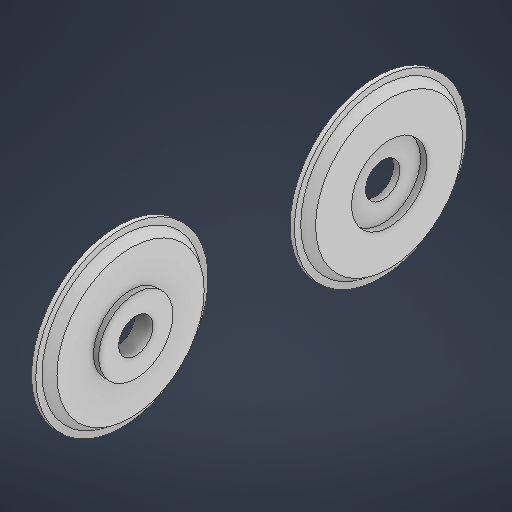
# Autodesk Inventor part: Polea_pulgar_falange1
Saved by Autodesk Inventor 2026.1 (Build 301233020, 233B)
## iProperties
Created: 2026-02-22
Part Number: Polea_pulgar_falange1
Material: Generic
Document SubType Name: Modeling
Designer: user
Density: 1 g/cm^3
Appearance: Default
Author: user
Autodesk Inventor part; units mm, degrees
ref_plane "XY Plane" through (0, 0, 0) normal (0, 0, 1) x (1, 0, 0)
sketch "Sketch1" plane through (0, 0, 0) normal (1, 0, 0) x (0, 1, 0)
  circle A0 centre (0, 0) radius 8.5399
  dimension "d0" = 17.0798
  constraints: 1 centre point, 1 coincident
  measures "d0" diameter of A0
extrude "Extrusion1" add sketch "Sketch1" along normal mid plane 2
sketch "Sketch2" plane through (-1, 0, 0) normal (-1, 0, 0) x (0, 0, 1)
  circle A0 centre (0, 0) radius 10
  dimension "d41" = 20
  constraints: 1 centre point, 1 coincident
  measures "d41" diameter of A0
extrude "Extrusion2" add sketch "Sketch2" along normal blind 0.5
sketch "Sketch3" plane through (-1.5, 0, 0) normal (-1, 0, 0) x (0, 0, 1)
  point P0 (0, 0)
sketch "Sketch5" plane through (0, 0, 0) normal (0, 1, 0) x (-1, 0, 0)
  circle A0 centre (0, -0.6447) radius 0.3263
  line L0 (-1.5, 0) -> (1.5, 0)
  circle A1 centre (0, 0.6447) radius 0.3263
  point P0 (0, 0)
  constraints: 2 centre point, 2 end point, 1 symmetric about line, 1 other
sketch "Sketch6" plane through (0, 0, 0) normal (0, 1, 0) x (-1, 0, 0)
  line L0 (1, -8.5399) -> (1, 8.5399) projected
  line L1 (1, -8.5399) -> (-1, -8.5399) projected
  line L2 (0, -8.5399) -> (1, -5.5929)
  line L3 (1, -10) -> (1, 10) projected
  line L4 (0, -8.5399) -> (-1, -9.2623)
  line L5 (-1, -9.2623) -> (-1, -8.5399)
  line L6 (1, -8.5399) -> (1, -9.2623)
  line L7 (-2.6263, 0) -> (3.0126, 0)
  line L8 (-1, -9.2623) -> (-1, -8.5399)
  line L9 (0, -8.5399) -> (1, -8.5399)
  point P0 (0, 0)
  constraints: 14 end point, 1 horizontal, 1 midpoint, 1 perpendicular, 1 point on line
revolve "Revolution1" add sketch "Sketch6" angle 360 about axis through (2.6263, 0, 0) along (-1, 0, 0) contours L4 L5 L1
mirror "Mirror3" about plane through (0, 0, 0) normal (1, 0, 0) of "Revolution1"
sketch "Sketch7" plane through (0, 0, 0) normal (0, 1, 0) x (-1, 0, 0)
  line L0 (-5.9098, -10.3165) -> (0, -10.3165)
  line L1 (0, -10.3165) -> (0, 11.166)
  line L2 (0, 11.166) -> (-5.9098, 11.166)
  line L3 (-5.9098, 11.166) -> (-5.9098, -10.3165)
  point P0 (0, 0)
  constraints: 8 end point, 2 parallel, 1 horizontal, 1 perpendicular
extrude "Extrusion6" cut sketch "Sketch7" along normal mid plane 24.5
sketch "Sketch8" plane through (0, 0, 0) normal (1, 0, 0) x (0, 1, 0)
  circle A0 centre (0, 0) radius 2
  dimension "d15" = 4
  constraints: 1 centre point, 1 coincident
  measures "d15" diameter of A0
extrude "Extrusion7" cut sketch "Sketch8" against normal through all
sketch "Sketch9" plane through (0, 0, 0) normal (1, 0, 0) x (0, 0, -1)
  circle A0 centre (0, 0) radius 4.374
  line L0 (1.4796, -4.1161) -> (1.4796, -1.3457)
  circle A1 centre (0, 0) radius 2 projected
  arc A2 (1.4796, -1.3457) -> (-1.4796, -1.3457) centre (0, 0) ccw
  line L1 (0.971, -8.4845) -> (0.971, 2) projected
  line L2 (-1.4796, -4.1161) -> (-1.4796, -1.3457)
  line L3 (-0.971, 2) -> (-0.971, -8.4845) projected
  point P0 (0.971, -4.7727)
  point P1 (0, 2)
  point P2 (0, 2)
  point P3 (-0.971, -4.7727)
  point P4 (-1.4796, -1.3457)
  point P5 (0.971, -7.875)
  point P6 (-0.971, -7.875)
  dimension "d22" = 0.5086
  dimension "d23" = 0.5086
  dimension "d36" = 8.7479
  constraints: 5 point on circle, 4 end point, 2 centre point, 2 coincident, 1 parallel, 1 vertical, 2 other
  measures "d36" diameter of A0
extrude "Extrusion8" cut sketch "Sketch9" against normal blind 0.75 contours A0 L0 A1 L2 | L2 A1 L3 A0 | A0 L1 A1 L0 | L3 A1 L1 A0
pattern_linear "Rectangular Pattern3" count 2 spacing 30 along (0, 0, 1) of "Extrusion1", "Extrusion2", "Revolution1", "Extrusion6", "Extrusion7", "Mirror3"
sketch "Sketch10" plane through (0, -4.7727, 20.971) normal (1, 0, 0) x (0, 0, -1)
  arc A0 (-9.029, 6.7727) -> (-9.029, 6.7727) centre (-9.029, 4.7727) ccw projected
  circle A1 centre (-9.029, 4.7727) radius 2
  circle A2 centre (-9.029, 4.7727) radius 4.299
  point P0 (20.971, 4.7727)
  point P1 (1.942, 0)
  point P2 (0, 0)
  dimension "d44" = 8.5979
  constraints: 2 centre point, 2 coincident, 1 concentric
  measures "d44" diameter of A2
extrude "Extrusion9" add sketch "Sketch10" along normal blind 0.6
sketch "Sketch11" plane through (0, 0, 0) normal (1, 0, 0) x (0, 0, 1)
  line L0 (-15.9707, 13.7758) -> (17.9357, 13.7758)
  line L1 (17.9357, 13.7758) -> (17.9357, -12.8142)
  line L2 (17.9357, -12.8142) -> (-15.9707, -12.8142)
  line L3 (-15.9707, -12.8142) -> (-15.9707, 13.7758)
  point P0 (0, 0)
  constraints: 8 end point, 2 parallel, 1 horizontal, 1 perpendicular
ref_plane "Work Plane7" through (0, 0, 30) normal (1, 0, 0) x (0, 1, 0)
equation "\"tolerancia\" = 0.15"
body "Solid1"
